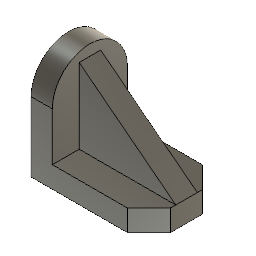
A1 HomeWork2 (Autodesk Fusion 360 design; units mm, degrees)
Autodesk Fusion 360 part; units mm, degrees
sketch "Sketch1" plane through (0, 0, 0) normal (0, 0, 1) x (1, 0, 0)
  line L0 (0, 42) -> (0, 0)
  line L1 (66, 12) -> (54, 0)
  line L2 (0, 0) -> (54, 0)
  line L3 (54, 42) -> (66, 30)
  line L4 (66, 30) -> (66, 12)
  line L5 (0, 42) -> (54, 42)
  constraint vertical L0
  constraint coincident L0.end L2.start
  constraint perpendicular L0 L2
  constraint perpendicular L0 L5
extrude "Extrude1" add sketch "Sketch1" along normal blind 12
sketch "Sketch2" plane through (0, 0, 12) normal (0, 0, 1) x (-1, 0, 0)
  line L0 (0, 0) -> (-54, 0)
  line L1 (-54, 0) -> (-66, -12)
  line L2 (-66, -12) -> (-66, -30)
  line L3 (-66, -30) -> (-54, -42)
  line L4 (-54, -42) -> (0, -42)
  line L5 (0, -42) -> (0, 0)
  line L6 (0, -42) -> (-12, -42)
  line L7 (-12, -42) -> (-12, 0)
  line L8 (-12, 0) -> (0, 0)
  line L9 (0, 0) -> (0, -42)
  dimension "d9" = 12
  constraint horizontal L6
  constraint vertical L7
  constraint horizontal L8
  constraint vertical L9
  constraint coincident L0 L7.end
  constraint coincident L4.end L5.start
  measures "d9" distance of L7 L9
extrude "Extrude2" add sketch "Sketch2" along normal blind 27 contours L0 L4 L5 L6 L7 L8 L9
sketch "Sketch3" plane through (0, 0, 12) normal (0, 0, 1) x (-1, 0, 0)
  line L0 (-12, -42) -> (-12, 0)
  line L1 (-12, 0) -> (-54, 0)
  line L2 (-54, 0) -> (-66, -12)
  line L3 (-66, -12) -> (-66, -30)
  line L4 (-66, -30) -> (-54, -42)
  line L5 (-54, -42) -> (-12, -42)
  line L6 (-12, 0) -> (-12, -15)
  line L7 (-12, -15) -> (-66, -15)
  line L8 (-12, -15) -> (-12, -27)
  line L9 (-12, -27) -> (-66, -27)
  line L10 (-66, -15) -> (-66, -27)
  dimension "d12" = 15
  dimension "d14" = 12
  constraint coincident L0.end L1.start
  constraint perpendicular L1 L6
  constraint coincident L3 L7.end
  constraint perpendicular L3 L7
  constraint perpendicular L7 L8
  constraint coincident L3 L9.end
  constraint perpendicular L3 L9
  measures "d12" distance of L0.end L6.end
  measures "d14" distance of L6.end L8.end
extrude "Extrude3" add sketch "Sketch3" along normal blind 42 contours L0 L3 L7 L8 L9 L10
sketch "Sketch5" plane through (0, 15, 0) normal (0, -1, 0) x (1, 0, 0)
  line L0 (12, 12) -> (66, 12)
  line L1 (66, 12) -> (66, 54)
  line L2 (66, 54) -> (12, 54)
  line L3 (12, 54) -> (12, 39)
  line L4 (12, 39) -> (12, 12)
  line L5 (12, 54) -> (66, 12)
  line L6 (12, 54) -> (66, 54)
  line L7 (66, 54) -> (66, 12)
  constraint coincident L2.end L3.start
  constraint coincident L0.end L1.start
  constraint coincident L1.end L2.start
extrude "Extrude4" cut sketch "Sketch5" against normal blind 12 contours L1 L2 L5 L6 L7
sketch "Sketch6" plane through (0, 0, 0) normal (-1, 0, 0) x (0, -1, 0)
  line L0 (-42, 0) -> (0, 0)
  line L1 (0, 0) -> (0, 39)
  line L2 (0, 39) -> (-42, 39)
  line L3 (-42, 39) -> (-42, 0)
  circle A0 centre (-21, 39) radius 21
  line L4 (-42, 39) -> (0, 39)
  dimension "d19" = 42
  constraint midpoint L2 A0.centre
  constraint coincident L2.end L3.start
  constraint coincident L1.end L2.start
  measures "d19" diameter of A0
extrude "Extrude5" add sketch "Sketch6" against normal blind 12 contours L2 A0 L4 picked at (-14.615, 43.0805)
